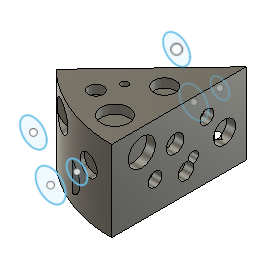
Kaese v1 (Autodesk Fusion 360 design; units mm, degrees)
Autodesk Fusion 360 part; units mm, degrees
note: some values were not read from the file. Set by a fixed rule: which sketch regions a step uses.
sketch "Skizze1" plane through (0, 0, 0) normal (0, 1, 0) x (1, 0, 0)
  line L0 (0, 0) -> (0, -15)
  line L1 (0, -15) -> (15, -15)
  line L2 (15, -15) -> (15, 0)
  line L3 (15, 0) -> (0, 0)
  line L4 (15, 0) -> (17.5, 0)
  line L5 (17.5, 0) -> (17.5, -15)
  line L6 (17.5, -15) -> (15, -15)
  dimension "d1" = 15
  dimension "d2" = 15
  dimension "d3" = 2.5
  constraint coincident L0.start L3.end
  constraint vertical L0
  constraint perpendicular L0 L1
  constraint perpendicular L1 L2
  constraint perpendicular L0 L3
  constraint perpendicular L2 L4
  constraint perpendicular L3 L5
  constraint perpendicular L2 L6
  measures "d1" distance of L0.start L0.end
  measures "d2" distance of L0.end L1.end
  measures "d3" distance of L2.end L4.end
sketch "Skizze2" plane through (0, 13, 0) normal (0, 1, 0) x (-1, 0, 0)
sketch "Skizze3" plane through (0, 0, 0) normal (0, 1, 0) x (1, 0, 0)
  line L0 (0, 0) -> (0, -15)
  line L1 (0, -15) -> (0, 0)
  circle A0 centre (0, 0) radius 15
  line L2 (0, 0) -> (-10.3643, -10.8435)
  constraint coincident L0.start L1.end
  constraint vertical L0
  constraint parallel L0 L1
  constraint coincident A0 L2.end
extrude "Extrusion2" add sketch "Skizze3" along normal blind 9 contours L0 L1 A0 L2 picked at (-1.8916, -9.7989)
sketch "Skizze4" plane through (0, 0, 0) normal (-0.722902, 0, -0.690951) x (-0.690951, 0, 0.722902)
  line L0 (0, 0) -> (15, 0)
  line L1 (15, 0) -> (15, 9)
  line L2 (15, 9) -> (0, 9)
  line L3 (0, 9) -> (0, 0)
  circle A0 centre (2.6906, 2.7068) radius 0.759
  circle A1 centre (3.9712, 6.7561) radius 1.6237
  circle A2 centre (11.6545, 6.7561) radius 1.1059
  circle A3 centre (7.6744, 3.9181) radius 0.5299
  circle A4 centre (7.6744, 6.7561) radius 0.6239
  circle A5 centre (9, 1.5) radius 0.8703
  circle A6 centre (11.7237, 4.0566) radius 1.4228
extrude "Extrusion3" cut sketch "Skizze4" against normal blind 1 contours A0 | A1 | A2 | A3 | A4 | A5 | A6
sketch "Skizze5" plane through (0, 9, 0) normal (0, 1, 0) x (-1, 0, 0)
  line L0 (0, 0) -> (10.3643, 10.8435)
  arc A0 (10.3643, 10.8435) -> (0, 15) centre (0, 0) ccw
  line L1 (0, 15) -> (0, 0)
  circle A1 centre (2.6465, 11.993) radius 1.5376
  circle A2 centre (2.6465, 6.4536) radius 1.1912
  circle A3 centre (6.1213, 10.6395) radius 0.8189
  circle A4 centre (5.1094, 8.4518) radius 0.4
extrude "Extrusion4" cut sketch "Skizze5" against normal blind 1 contours A1 | A2 | A3 | A4
sketch "Skizze6" plane through (0, 0, 0) normal (1, 0, 0) x (0, 0, -1)
  line L0 (-15, 0) -> (0, 0)
  line L1 (0, 0) -> (0, 9)
  line L2 (0, 9) -> (-15, 9)
  line L3 (-15, 9) -> (-15, 0)
  circle A0 centre (-11.6448, 6.5689) radius 1.5047
  circle A1 centre (-10.1749, 3.2155) radius 0.7721
  circle A2 centre (-4.3869, 6.3622) radius 0.7676
  circle A3 centre (-5.9028, 3.2155) radius 0.5958
  circle A4 centre (-2.4117, 3.9046) radius 1.2257
  circle A5 centre (-7.924, 5.5353) radius 0.9866
  circle A6 centre (-6.7297, 2.2968) radius 0.8791
extrude "Extrusion5" cut sketch "Skizze6" against normal blind 1 contours A0 | A1 | A2 | A3 A6 | A3 A6 | A3 A6 | A4 | A5
sketch "Skizze7" plane through (0, 0, 0) normal (0, 0, 1) x (1, 0, 0)
  circle A0 centre (-7.7636, 6.803) radius 1.5064
  circle A1 centre (-2.9408, 5.4698) radius 1.0472
  circle A2 centre (-5.8227, 2.6859) radius 1.6102
ref_plane "Arbeitsebene1" through (-7.7636, 6.803, 16) normal (0, 0, 1) x (1, 0, 0)
sketch "Skizze8" plane through (0, 0, 16) normal (0, 0, 1) x (1, 0, 0)
  circle A0 centre (-7.7283, 6.7967) radius 1.4872
  circle A1 centre (-5.8039, 2.6728) radius 1.6738
  circle A2 centre (-2.8714, 5.4221) radius 1.1553
extrude "Extrusion6" cut sketch "Skizze8" against normal blind 2
extrude "Extrusion7" cut sketch "Skizze8" against normal blind 4 contours A0
sketch "Skizze9" plane through (0, 0, 0) normal (0, -1, 0) x (1, 0, 0)
  line L0 (-10.3643, 10.8435) -> (0, 0)
  line L1 (0, 0) -> (0, 15)
  arc A0 (0, 15) -> (-10.3643, 10.8435) centre (0, 0) ccw
  line L2 (0, 0) -> (-5.5833, 13.9222)
  circle A1 centre (-4.3092, 10.7452) radius 1.85
  dimension "d19" = 3.7
  constraint coincident L0.end L1.start
  constraint midpoint A0 L2.end
  constraint coincident L2 A1.centre
  measures "d19" diameter of A1
extrude "Extrusion8" cut sketch "Skizze9" against normal blind 7 contours L2 A1 | L2 A1
